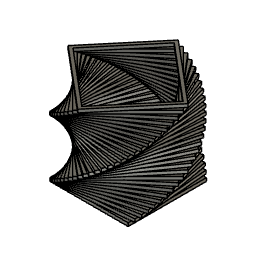
spin_box (Autodesk Fusion 360 design; units mm, degrees)
Autodesk Fusion 360 part; units mm, degrees
sketch "Sketch1" plane through (0, 0, 0) normal (0, 0, 1) x (1, 0, 0)
  line L0 (-58.6676, 55.9345) -> (63.8324, 55.9345)
  line L1 (63.8324, 55.9345) -> (63.8324, -66.5655)
  line L2 (63.8324, -66.5655) -> (-58.6676, -66.5655)
  line L3 (-58.6676, -66.5655) -> (-58.6676, 55.9345)
  line L4 (58.8324, -61.5655) -> (-53.6676, -61.5655)
  line L5 (-53.6676, -61.5655) -> (-53.6676, 50.9345)
  line L6 (-53.6676, 50.9345) -> (58.8324, 50.9345)
  line L7 (58.8324, 50.9345) -> (58.8324, -61.5655)
  line L8 (-58.6676, -5.3155) -> (63.8324, -5.3155)
  line L9 (2.5824, 55.9345) -> (2.5824, 50.9345)
  line L10 (2.5824, -61.5655) -> (2.5824, -66.5655)
  line L11 (2.5824, 50.9345) -> (2.5824, -61.5655)
  point P0 (2.5824, 55.9345)
  point P1 (-58.6676, -5.3155)
  point P2 (2.5824, -66.5655)
  point P3 (63.8324, -5.3155)
  point P4 (58.8324, -5.3155)
  point P5 (-53.6676, -5.3155)
  point P6 (2.5824, 50.9345)
  point P7 (2.5824, -61.5655)
  point P8 (2.5824, -5.3155)
  dimension "d9" = 122.5
  dimension "d10" = 122.5
  dimension "d11" = 5
  constraint horizontal L0
  constraint vertical L1
  constraint horizontal L2
  constraint vertical L3
  constraint midpoint L0 P0
  constraint midpoint L3 P1
  constraint midpoint L2 P2
  constraint midpoint L1 P3
  constraint midpoint L7 P4
  constraint midpoint L5 P5
  constraint midpoint L6 P6
  constraint midpoint L4 P7
  constraint coincident P1 L8.start
  constraint coincident P3 L8.end
  constraint coincident P0 L9.start
  constraint coincident P6 L9.end
  constraint coincident P7 L10.start
  constraint coincident P2 L10.end
  constraint midpoint L8 P8
  measures "d9" distance of L0.start L0.end
  measures "d10" distance of L0.start L2.end
extrude "Extrude1" add sketch "Sketch1" along normal blind 5 contours L5 L6 L8 L11 | L6 L7 L8 L11 | L4 L5 L8 L11 | L4 L7 L8 L11 makes body 1
extrude "Extrude3" add sketch "Sketch1" along normal blind 5 separate body contours L0 L3 L5 L6 L8 L9 | L0 L1 L6 L7 L8 L9 | L2 L3 L4 L5 L8 L10 | L1 L2 L4 L7 L8 L10 makes body 2
copy_body "CopyPasteBodies8" bodies 2 makes body 3
move_body "Move7" bodies 3 to x (0.996195, 0.087156, 0) y (-0.087156, 0.996195, 0) z (0, 0, 1) at (-0.4714, -0.2633, 5)
copy_body "CopyPasteBodies9" bodies 3 2 makes body 4 makes body 5
move_body "Move8" bodies 4 5 to x (0.984808, 0.173648, 0) y (-0.173648, 0.984808, 0) z (0, 0, 1) at (-0.918, -0.5667, 10)
copy_body "CopyPasteBodies10" bodies 5 3 2 4 makes body 6 makes body 7 makes body 8 makes body 9
move_body "Move9" bodies 6 7 8 9 to x (0.939693, 0.34202, 0) y (-0.34202, 0.939693, 0) z (0, 0, 1) at (-1.7237, -1.2842, 20)
copy_body "CopyPasteBodies11" bodies 9 3 2 5 7 8 4 6 makes body 10 makes body 11 makes body 12 makes body 13 makes body 14 makes body 15 makes body 16 makes body 17
move_body "Move10" bodies 10 11 12 13 14 15 16 17 to x (0.766044, 0.642788, 0) y (-0.642788, 0.766044, 0) z (0, 0, 1) at (-2.9042, -3.0805, 40)
copy_body "CopyPasteBodies12" bodies 17 16 makes body 18 makes body 19
copy_body "CopyPasteBodies13" bodies 10 18 makes body 20 makes body 21
move_body "Move11" bodies 20 21 to x (0.984808, 0.173648, 0) y (-0.173648, 0.984808, 0) z (0, 0, 1) at (-0.918, -0.5667, 10)
copy_body "CopyPasteBodies14" bodies 21 3 2 5 7 9 8 16 12 17 14 20 15 19 13 18 10 4 11 6 makes body 22 makes body 23 makes body 24 makes body 25 makes body 26 makes body 27 makes body 28 makes body 29 makes body 30 makes body 31 makes body 32 makes body 33 makes body 34 makes body 35 makes body 36 makes body 37 makes body 38 makes body 39 makes body 40 makes body 41
move_body "Move12" bodies 22 23 24 25 26 27 28 29 30 31 32 33 34 35 36 37 38 39 40 41 to x (0, 1, 0) y (-1, 0, 0) z (0, 0, 1) at (-2.7501, -8.3096, 90)
ref_plane "WorkPlane1" through (89.0842, 1.7286, 145) normal (0, 0, 1) x (1, 0, 0)
combine "Combine1" operation add target body 1 tool bodies 14 6 19 20 21 2 11 12 5 8 9 3 4 18 10 7 13 15 17 23 24 25 26 16 35 27 33 29 28 39 37 34 41 32 30 31 38 40 36 22
split "Split1" by plane through (89.0842, 1.7286, 145) normal (0, 0, 1) bodies 1 makes body 42 at (60.6801, -29.6322, 180)
copy_body "Body->Comp1" bodies 1 removing the originals makes body 43 in component "Component"
component "Component" placed x (1, 0, 0) y (0, 1, 0) z (0, 0, 1) at (0, 0, 0)
hidden bodies 42
equation "shelfdepth = 25.5 cm"
equation "mintteabagwidth = 75 mm"
equation "mintteabagheight = 75.7 mm"
equation "herbaltea2width = 129.54 mm"
equation "herbalteaheight = 68.4 mm"
equation "boxheight = 55.5 mm"
equation "thickness = 5 mm"
equation "give = 15 mm"
equation "d9 = ( 1.5 * mintteabagwidth ) + ( 2 * thickness )"
equation "d10 = ( 1.5 * mintteabagwidth ) + ( 2 * thickness )"
equation "d11 = thickness"
equation "d12 = thickness"
equation "d16 = thickness"
equation "angle = 5 deg"
